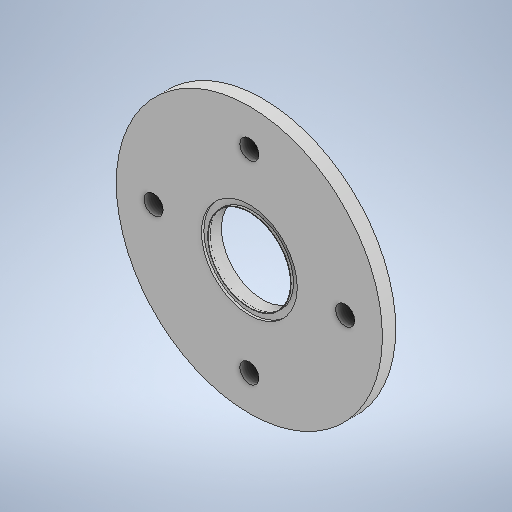
# Autodesk Inventor part: pięćśetka
Saved by Autodesk Inventor 2025 (Build 290162000, 162)
## iProperties
Created: 2025-05-19
Part Number: pięćśetka
Material: Ogólny
Document SubType Name: Modeling
Designer: failc
Density: 1 g/cm^3
Appearance: Domyślna
Author: failc
Autodesk Inventor part; units mm, degrees
ref_plane "YZ Plane" through (0, 0, 0) normal (1, 0, 0) x (0, 1, 0)
ref_plane "XZ Plane" through (0, 0, 0) normal (0, 1, 0) x (-1, 0, 0)
ref_plane "XY Plane" through (0, 0, 0) normal (0, 0, 1) x (1, 0, 0)
sketch "Szkic1" plane through (0, 0, 0) normal (0, 0, 1) x (1, 0, 0)
  circle A0 centre (0, 0) radius 250
  dimension "d0" = 500
  constraints: 1 centre point, 1 coincident
  measures "d0" diameter of A0
extrude "Wyciągnięcie proste1" add sketch "Szkic1" along normal blind 25
sketch "Szkic2" plane through (0, 0, 25) normal (0, 0, 1) x (1, 0, 0)
  circle A0 centre (0, 180) radius 18
  circle A1 centre (180, 0) radius 18
  circle A2 centre (0, -184) radius 18
  circle A3 centre (-180, 0) radius 18
  point P0 (0, 0)
  dimension "d3" = 36
  dimension "d4" = 36
  dimension "d5" = 36
  dimension "d6" = 36
  constraints: 4 centre point
  measures "d3" diameter of A0
  measures "d4" diameter of A1
  measures "d5" diameter of A2
  measures "d6" diameter of A3
extrude "Wyciągnięcie proste2" cut sketch "Szkic2" against normal blind 25
thread "Gwint1" size "M36x4" class "6H" standard "ANSI Metric M Profile" full length
thread "Gwint2" size "M36x4" class "6H" standard "ANSI Metric M Profile" full length
thread "Gwint3" size "M36x4" class "6H" standard "ANSI Metric M Profile" full length
thread "Gwint4" size "M36x4" class "6H" standard "ANSI Metric M Profile" full length
sketch "Szkic3" plane through (0, 0, 25) normal (0, 0, 1) x (1, 0, 0)
  circle A0 centre (0, 0) radius 85
  dimension "d17" = 170
  constraints: 1 centre point, 1 coincident
  measures "d17" diameter of A0
extrude "Wyciągnięcie proste3" cut sketch "Szkic3" against normal blind 200
sketch "Szkic4" plane through (0, 0, 25) normal (0, 0, 1) x (1, 0, 0)
  circle A0 centre (0, 0) radius 77.5
  dimension "d20" = 155
  constraints: 1 centre point, 1 coincident
  measures "d20" diameter of A0
sketch "Szkic5" plane through (0, 0, 25) normal (0, 0, 1) x (1, 0, 0)
  circle A0 centre (0, 0) radius 85
  dimension "d21" = 170
  constraints: 1 centre point, 1 coincident
  measures "d21" diameter of A0
extrude "Wyciągnięcie proste4" add sketch "Szkic5" against normal blind 25
extrude "Wyciągnięcie proste5" cut sketch "Szkic4" against normal blind 25
sketch "Szkic6" plane through (0, 0, 25) normal (0, 0, 1) x (1, 0, 0)
  circle A0 centre (0, 0) radius 82
  circle A1 centre (0, 0) radius 87
  dimension "d26" = 164
  dimension "d27" = 174
  constraints: 2 centre point, 2 coincident
  measures "d26" diameter of A0
  measures "d27" diameter of A1
extrude "Wyciągnięcie proste6" cut sketch "Szkic6" against normal blind 4.5
sketch "Szkic7" plane through (0, 0, 25) normal (0, 0, 1) x (1, 0, 0)
  circle A0 centre (0, 0) radius 79.5
  circle A1 centre (0, 0) radius 84.5
  dimension "d30" = 159
  dimension "d31" = 169
  constraints: 2 centre point, 2 coincident
  measures "d30" diameter of A0
  measures "d31" diameter of A1
extrude "Wyciągnięcie proste7" cut sketch "Szkic7" against normal blind 4.5
sketch "Szkic8" plane through (0, 0, 25) normal (0, 0, 1) x (1, 0, 0)
  circle A0 centre (0, 0) radius 78.5
  circle A1 centre (0, 0) radius 90
  dimension "d34" = 157
  dimension "d36" = 180
  constraints: 2 centre point, 1 coincident
  measures "d34" diameter of A0
  measures "d36" diameter of A1
extrude "Wyciągnięcie proste8" cut sketch "Szkic8" against normal blind 4.5
